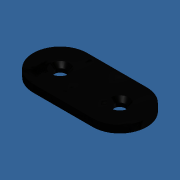
# Autodesk Inventor part: arm-top
Saved by Autodesk Inventor 2015 (Build 190159000, 159)
## iProperties
Created: 2019-01-20
Part Number: arm-top
Material: Generic
Document SubType Name: Modeling
Designer: gabriel
Density: 1 g/cm^3
Appearance: Default
Author: gabriel
Autodesk Inventor part; units mm, degrees
ref_plane "YZ Plane" through (0, 0, 0) normal (1, 0, 0) x (0, 1, 0)
ref_plane "XZ Plane" through (0, 0, 0) normal (0, 1, 0) x (-1, 0, 0)
ref_plane "XY Plane" through (0, 0, 0) normal (0, 0, 1) x (1, 0, 0)
sketch "Sketch36" plane through (0, 0, 0) normal (0, 0, 1) x (1, 0, 0)
  arc A0 (0, -5.7547) -> (0, 5.7547) centre (0, 0) ccw
  arc A1 (-12.7, 5.7547) -> (-12.7, -5.7547) centre (-12.7, 0) ccw
  line L0 (-12.7, 5.7547) -> (0, 5.7547)
  line L1 (-12.7, -5.7547) -> (0, -5.7547)
  circle A2 centre (-12.7, 0) radius 1.1906
  circle A3 centre (0, 0) radius 1.1906
  dimension "d158" = 11.5094
  dimension "d160" = 12.7
  dimension "d162" = 2.3813
  dimension "d163" = 2.3813
  dimension "d176" = 5.7547
  constraints: 4 centre point, 4 end point, 4 point on circle, 3 coincident, 2 parallel, 1 horizontal, 1 horizontal alignment, 1 tangent
  measures "d158" diameter of A0
  measures "d160" distance of point (0, 0) A1.centre
  measures "d162" diameter of A2
  measures "d163" diameter of A3
  measures "d176" radius of A1
extrude "Extrusion36" add sketch "Sketch36" along normal blind 1.5875
chamfer "Chamfer2" distance 0.7937 angle 45 2 edges at (-13.8906, 0, 1.5875) (-1.1906, 0, 1.5875)
body "Solid7"
